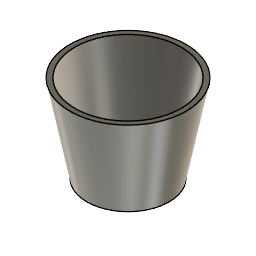
Emsamble (Autodesk Fusion 360 archive; units mm, degrees)
design "Maceta modelo"
Autodesk Fusion 360 part; units mm, degrees
sketch "Boceto1" plane through (0, 0, 0) normal (0, 0, 1) x (1, 0, 0)
  circle A0 centre (0, 0) radius 42.5
  dimension "d1" = 85
  constraint coincident A0.centre origin
  measures "d1" diameter of A0
ref_plane "PlanoDeObra1" through (0, 0, 90) normal (0, 0, 1) x (1, 0, 0)
sketch "Boceto2" plane through (0, 0, 90) normal (0, 0, 1) x (1, 0, 0)
  circle A0 centre (0, 0) radius 60
  dimension "d3" = 120
  constraint coincident A0.centre origin
  measures "d3" diameter of A0
loft "Solevación1" add profiles "Boceto1", "Boceto2" section 1 section 2
shell "Vaciado1" thickness 5 removed faces 1 at (14.661, 13.6035, 90)
